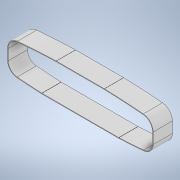
# Autodesk Inventor part: 7 Segment Clock Shell
Saved by Autodesk Inventor 2021 (Build 250183000, 183)
## iProperties
Created: 2020-06-27
Part Number: 7 Segment Clock Shell
Material: Generic
Document SubType Name: Modeling
Designer: dech3
Density: 1 g/cm^3
Appearance: Default
Author: dech3
Autodesk Inventor part; units mm, degrees
ref_plane "YZ Plane" through (0, 0, 0) normal (1, 0, 0) x (0, 1, 0)
ref_plane "XZ Plane" through (0, 0, 0) normal (0, 1, 0) x (-1, 0, 0)
ref_plane "XY Plane" through (0, 0, 0) normal (0, 0, 1) x (1, 0, 0)
sketch "Block1" plane through (0, 0, 0) normal (0, 0, 1) x (1, 0, 0)
  arc A0 (261.5609, 58.5131) -> (100.3256, 67.9894) centre (0, -3015.4231) ccw
  arc A1 (-100.3256, 67.9894) -> (-261.5609, 58.5131) centre (0, -3015.4231) ccw
  line L0 (-159.5034, -75) -> (159.5034, -75)
  arc A2 (-263.2612, -68.2167) -> (-160.4975, -74.9753) centre (0, 3150) ccw
  arc A3 (160.4975, -74.9753) -> (263.2612, -68.2167) centre (0, 3150) ccw
  arc A4 (300, 16.6643) -> (261.5609, 58.5131) centre (258, 16.6643) ccw
  arc A5 (263.2612, -68.2167) -> (300, -28.3498) centre (260, -28.3498) ccw
  arc A6 (-300, -28.3498) -> (-263.2612, -68.2167) centre (-260, -28.3498) ccw
  arc A7 (-261.5609, 58.5131) -> (-300, 16.6643) centre (-258, 16.6643) ccw
  arc A8 (-99.6752, 68) -> (-100.3256, 67.9894) centre (-99.6752, 48) ccw
  arc A9 (100.3256, 67.9894) -> (99.6752, 68) centre (99.6752, 48) ccw
  arc A10 (159.5034, -75) -> (160.4975, -74.9753) centre (159.5034, -55) ccw
  arc A11 (-160.4975, -74.9753) -> (-159.5034, -75) centre (-159.5034, -55) ccw
  line L1 (-99.6752, 68) -> (99.6752, 68)
  line L2 (300, 16.6643) -> (300, -28.3498)
  line L3 (-300, -28.3498) -> (-300, 16.6643)
  point P0 (0, -2.2582)
  point P1 (-300, 55)
  point P2 (300, 55)
  point P3 (-300, -65)
  point P4 (300, -65)
  point P5 (-160, -75)
  point P6 (160, -75)
  point P7 (-100, 68)
  point P8 (100, 68)
  dimension "d0" = 600
  dimension "d14" = 120
  dimension "d13" = 120
  dimension "d12" = 140
  dimension "d10" = 140
  dimension "d3" = 200
  dimension "d1" = 200
  dimension "d20" = 200
  dimension "d21" = 320
  dimension "d2" = 143
  dimension "d11" = 10
  dimension "d9" = 10
  dimension "d22" = 13
  dimension "d23" = 13
  dimension "d8" = 42
  dimension "d7" = 40
  dimension "d6" = 40
  dimension "d5" = 42
  dimension "d4" = 20
  measures "d0" distance between parallel lines of L2 L3
  measures "d14" distance of point (-300, 55) point (-300, -65)
  measures "d13" distance of point (300, 55) point (300, -65)
  measures "d12" horizontal distance of point (-300, -65) point (-160, -75)
  measures "d10" horizontal distance of point (300, -65) point (160, -75)
  measures "d3" horizontal distance of point (-300, 55) point (-100, 68)
  measures "d1" horizontal distance of point (300, 55) point (100, 68)
  measures "d20" distance of point (100, 68) point (-100, 68)
  measures "d21" distance of point (160, -75) point (-160, -75)
  measures "d2" distance from line of L0 point (-100, 68)
  measures "d11" vertical distance of point (-300, -65) point (-160, -75)
  measures "d9" vertical distance of point (300, -65) point (160, -75)
  measures "d22" vertical distance of point (100, 68) point (300, 55)
  measures "d23" vertical distance of point (-100, 68) point (-300, 55)
  measures "d8" radius of A4
  measures "d7" radius of A5
  measures "d6" radius of A6
  measures "d5" radius of A7
  measures "d4" radius of A8
sketch "Sketch2" plane through (0, 0, 0) normal (0, 0, 1) x (1, 0, 0)
  arc A0 (97.0768, 307.8268) -> (-64.1585, 317.3031) centre (-164.4841, -2766.1094) ccw
  arc A1 (-264.8098, 317.3031) -> (-426.045, 307.8268) centre (-164.4841, -2766.1094) ccw
  line L0 (-323.9875, 174.3137) -> (-4.9807, 174.3137)
  arc A2 (-427.7454, 181.097) -> (-324.9816, 174.3384) centre (-164.4841, 3399.3137) ccw
  arc A3 (-3.9866, 174.3384) -> (98.7771, 181.097) centre (-164.4841, 3399.3137) ccw
  arc A4 (135.5159, 265.9781) -> (97.0768, 307.8268) centre (93.5159, 265.9781) ccw
  arc A5 (98.7771, 181.097) -> (135.5159, 220.9639) centre (95.5159, 220.9639) ccw
  arc A6 (-464.4841, 220.9639) -> (-427.7454, 181.097) centre (-424.4841, 220.9639) ccw
  arc A7 (-426.045, 307.8268) -> (-464.4841, 265.9781) centre (-422.4841, 265.9781) ccw
  arc A8 (-264.1594, 317.3137) -> (-264.8098, 317.3031) centre (-264.1594, 297.3137) ccw
  arc A9 (-64.1585, 317.3031) -> (-64.8089, 317.3137) centre (-64.8089, 297.3137) ccw
  arc A10 (-4.9807, 174.3137) -> (-3.9866, 174.3384) centre (-4.9807, 194.3137) ccw
  arc A11 (-324.9816, 174.3384) -> (-323.9875, 174.3137) centre (-323.9875, 194.3137) ccw
  line L1 (-264.1594, 317.3137) -> (-64.8089, 317.3137)
  line L2 (135.5159, 265.9781) -> (135.5159, 220.9639)
  line L3 (-464.4841, 220.9639) -> (-464.4841, 265.9781)
  arc A12 (-426.2994, 310.816) -> (-467.4841, 265.9781) centre (-422.4841, 265.9781) ccw
  arc A13 (-264.9073, 320.3016) -> (-426.2994, 310.816) centre (-164.4841, -2766.1094) ccw
  arc A14 (-264.1594, 320.3137) -> (-264.9073, 320.3016) centre (-264.1594, 297.3137) ccw
  line L4 (-264.1594, 320.3137) -> (-64.8089, 320.3137)
  arc A15 (-64.0609, 320.3016) -> (-64.8089, 320.3137) centre (-64.8089, 297.3137) ccw
  arc A16 (97.3311, 310.816) -> (-64.0609, 320.3016) centre (-164.4841, -2766.1094) ccw
  arc A17 (138.5159, 265.9781) -> (97.3311, 310.816) centre (93.5159, 265.9781) ccw
  line L5 (138.5159, 265.9781) -> (138.5159, 220.9639)
  arc A18 (99.0217, 178.107) -> (138.5159, 220.9639) centre (95.5159, 220.9639) ccw
  arc A19 (-3.8375, 171.3421) -> (99.0217, 178.107) centre (-164.4841, 3399.3137) ccw
  arc A20 (-4.9807, 171.3137) -> (-3.8375, 171.3421) centre (-4.9807, 194.3137) ccw
  line L6 (-4.9807, 171.3137) -> (-323.9875, 171.3137)
  arc A21 (-325.1307, 171.3421) -> (-323.9875, 171.3137) centre (-323.9875, 194.3137) ccw
  arc A22 (-427.9899, 178.107) -> (-325.1307, 171.3421) centre (-164.4841, 3399.3137) ccw
  arc A23 (-467.4841, 220.9639) -> (-427.9899, 178.107) centre (-424.4841, 220.9639) ccw
  line L7 (-467.4841, 220.9639) -> (-467.4841, 265.9781)
  point P0 (0, 0)
  point P1 (-464.4841, 304.3137)
  point P2 (135.5159, 304.3137)
  point P3 (-464.4841, 184.3137)
  point P4 (135.5159, 184.3137)
  point P5 (-324.4841, 174.3137)
  point P6 (-4.4841, 174.3137)
  point P7 (-264.4841, 317.3137)
  point P8 (-64.4841, 317.3137)
  dimension "d44" = 143
  dimension "d47" = 600
  dimension "d50" = 600
  dimension "d51" = 120
  dimension "d52" = 120
  dimension "d53" = 140
  dimension "d54" = 140
  dimension "d55" = 200
  dimension "d56" = 200
  dimension "d57" = 200
  dimension "d58" = 320
  dimension "d59" = 143
  dimension "d60" = 10
  dimension "d61" = 10
  dimension "d62" = 13
  dimension "d63" = 13
  dimension "d64" = 42
  dimension "d65" = 40
  dimension "d66" = 40
  dimension "d67" = 42
  dimension "d68" = 20
  dimension "d69" = 3
  constraints: 56 point on circle, 24 centre point, 16 end point, 16 tangent, 8 point on line, 3 equal radius, 2 horizontal, 2 parallel, 2 perpendicular, 15 other
  measures "d44" distance between parallel lines of L0 L1
  measures "d47" distance between parallel lines of L2 L3
  measures "d50" distance between parallel lines of L2 L3
  measures "d51" distance of point (-464.484, 304.314) point (-464.484, 184.314)
  measures "d52" distance of point (135.516, 304.314) point (135.516, 184.314)
  measures "d53" horizontal distance of point (-464.484, 184.314) point (-324.484, 174.314)
  measures "d54" horizontal distance of point (135.516, 184.314) point (-4.484, 174.314)
  measures "d55" horizontal distance of point (-464.484, 304.314) point (-264.484, 317.314)
  measures "d56" horizontal distance of point (135.516, 304.314) point (-64.484, 317.314)
  measures "d57" distance of point (-64.484, 317.314) point (-264.484, 317.314)
  measures "d58" distance of point (-4.484, 174.314) point (-324.484, 174.314)
  measures "d59" distance from line of L0 point (-264.484, 317.314)
  measures "d60" vertical distance of point (-464.484, 184.314) point (-324.484, 174.314)
  measures "d61" vertical distance of point (135.516, 184.314) point (-4.484, 174.314)
  measures "d62" vertical distance of point (-64.484, 317.314) point (135.516, 304.314)
  measures "d63" vertical distance of point (-264.484, 317.314) point (-464.484, 304.314)
  measures "d64" radius of A4
  measures "d65" radius of A5
  measures "d66" radius of A6
  measures "d67" radius of A7
  measures "d68" radius of A8
  measures "d69" radial gap between concentric circles of A7 A12
extrude "Extrusion2" add sketch "Sketch2" along normal blind 80
body "Solid2"
